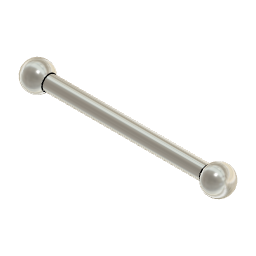
spindle v1 (Autodesk Fusion 360 design; units mm, degrees)
Autodesk Fusion 360 part; units mm, degrees
cylinder "CylinderPrimitive1" add diameter 8 height 100 placed x (0, 0, -1) y (0, 1, 0) z (1, 0, 0) at (0, 0, 0)
sphere "SpherePrimitive1" add diameter 15 placed x (0, -1, 0) y (0, 0, 1) z (-1, 0, 0) at (0, 0, 0)
sphere "SpherePrimitive2" add diameter 15 placed x (0, 1, 0) y (0, 0, 1) z (1, 0, 0) at (100, 0, 0)
